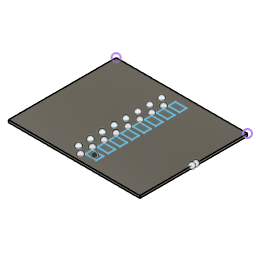
sequence (Autodesk Fusion 360 design; units mm, degrees)
Autodesk Fusion 360 part; units mm, degrees
box "BoxPrimitive1" add length 136 width 166 height 3 placed x (0, -1, 0) y (1, 0, 0) z (0, 0, 1) at (-30, 40, 0)
move_body "Move1" bodies 1 to x (1, 0, 0) y (0, 1, 0) z (0, 0, 1) at (-59.3373, 23.0424, 23.0424)
move_body "Move2" bodies 1 to x (1, 0, 0) y (0, 1, 0) z (0, 0, 1) at (6.3373, 4.9576, -26.0424)
move_body "Move3" bodies 1 to x (1, 0, 0) y (0, 1, 0) z (0, 0, 1) at (0, 0, 3)
sketch "Sketch6" plane through (0, 0, 3) normal (0, 0, 1) x (-1, 0, 0)
  line L0 (83, 68) -> (-83, 68)
  line L1 (-83, 68) -> (-83, -68)
  line L2 (83, -68) -> (83, 68)
  line L3 (11, 54) -> (9, 54)
  line L4 (9, 54) -> (9, 51)
  line L5 (9, 51) -> (11, 51)
  line L6 (11, 51) -> (11, 54)
  line L7 (11, 39) -> (9, 39)
  line L8 (11, 36) -> (11, 39)
  line L9 (9, 39) -> (9, 36)
  line L10 (9, 36) -> (11, 36)
  line L11 (11, 24) -> (9, 24)
  line L12 (11, 21) -> (11, 24)
  line L13 (9, 24) -> (9, 21)
  line L14 (9, 21) -> (11, 21)
  line L15 (11, 9) -> (9, 9)
  line L16 (11, 6) -> (11, 9)
  line L17 (9, 9) -> (9, 6)
  line L18 (9, 6) -> (11, 6)
  line L19 (11, -6) -> (9, -6)
  line L20 (11, -9) -> (11, -6)
  line L21 (9, -6) -> (9, -9)
  line L22 (9, -9) -> (11, -9)
  line L23 (11, -21) -> (9, -21)
  line L24 (11, -24) -> (11, -21)
  line L25 (9, -21) -> (9, -24)
  line L26 (9, -24) -> (11, -24)
  line L27 (11, -36) -> (9, -36)
  line L28 (11, -39) -> (11, -36)
  line L29 (9, -36) -> (9, -39)
  line L30 (9, -39) -> (11, -39)
  line L31 (11, -51) -> (9, -51)
  line L32 (11, -54) -> (11, -51)
  line L33 (9, -51) -> (9, -54)
  line L34 (9, -54) -> (11, -54)
  line L35 (-82, -2.7) -> (-83, -2.7)
  line L36 (-83, 2.3) -> (-82, 2.3)
  line L37 (-82, 2.3) -> (-82, -2.7)
  line L38 (-3, 48) -> (-17, 48)
  line L39 (-17, 48) -> (-17, 57)
  line L40 (-17, 57) -> (-3, 57)
  line L41 (-3, 57) -> (-3, 48)
  line L42 (-17, 42) -> (-3, 42)
  line L43 (-17, 33) -> (-17, 42)
  line L44 (-3, 42) -> (-3, 33)
  line L45 (-3, 33) -> (-17, 33)
  line L46 (-17, 27) -> (-3, 27)
  line L47 (-17, 18) -> (-17, 27)
  line L48 (-3, 27) -> (-3, 18)
  line L49 (-3, 18) -> (-17, 18)
  line L50 (-17, 12) -> (-3, 12)
  line L51 (-17, 3) -> (-17, 12)
  line L52 (-3, 12) -> (-3, 3)
  line L53 (-3, 3) -> (-17, 3)
  line L54 (-17, -3) -> (-3, -3)
  line L55 (-17, -12) -> (-17, -3)
  line L56 (-3, -3) -> (-3, -12)
  line L57 (-3, -12) -> (-17, -12)
  line L58 (-17, -18) -> (-3, -18)
  line L59 (-17, -27) -> (-17, -18)
  line L60 (-3, -18) -> (-3, -27)
  line L61 (-3, -27) -> (-17, -27)
  line L62 (-17, -33) -> (-3, -33)
  line L63 (-17, -42) -> (-17, -33)
  line L64 (-3, -33) -> (-3, -42)
  line L65 (-3, -42) -> (-17, -42)
  line L66 (-17, -48) -> (-3, -48)
  line L67 (-17, -57) -> (-17, -48)
  line L68 (-3, -48) -> (-3, -57)
  line L69 (-3, -57) -> (-17, -57)
  point P0 (0, 60)
  point P1 (10, 52.5)
  point P2 (-10, 52.5)
  point P3 (10, 37.5)
  point P4 (10, 22.5)
  point P5 (10, 7.5)
  point P6 (10, -7.5)
  point P7 (10, -22.5)
  point P8 (10, -37.5)
  point P9 (10, -52.5)
  point P10 (-10, 52.5)
  point P11 (0, 45)
  point P12 (0, 30)
  point P13 (0, 15)
  point P14 (0, -15)
  point P15 (0, -30)
  point P16 (0, -45)
  dimension "d41" = 3
  dimension "d50" = 5
  dimension "d51" = 14
  dimension "d52" = 9
  constraint horizontal L3
  constraint perpendicular L3 L4
  constraint parallel L3 L5
  constraint parallel L4 L6
  constraint horizontal L35
  constraint horizontal L36
  constraint vertical L37
  constraint horizontal L38
  constraint perpendicular L38 L39
  constraint parallel L38 L40
  constraint parallel L39 L41
  constraint coincident P10 P2
  measures "d41" distance of L3.end L4.end
  measures "d50" distance of L35.start L36.end
  measures "d51" distance of L39.end L40.end
  measures "d52" distance of L38.end L39.end
sketch "Sketch4" plane through (0, 0, 3) normal (0, 0, 1) x (-1, 0, 0)
  line L0 (83, 68) -> (-83, 68)
  line L1 (-83, 68) -> (-83, -68)
  line L2 (-83, -68) -> (83, -68)
  line L3 (83, -68) -> (83, 68)
  line L4 (0, 0) -> (0, -20)
  line L5 (0, 0) -> (0, 20)
  line L6 (0, 0) -> (-15, 0)
  line L7 (1, -18.5) -> (-1, -18.5)
  line L8 (-1, -18.5) -> (-1, -21.5)
  line L9 (-1, -21.5) -> (1, -21.5)
  line L10 (1, -21.5) -> (1, -18.5)
  line L11 (1, -18.5) -> (-1, -21.5) construction
  line L12 (-1, -18.5) -> (1, -21.5) construction
  line L13 (-1, 18.5) -> (1, 18.5)
  line L14 (1, 18.5) -> (1, 21.5)
  line L15 (1, 21.5) -> (-1, 21.5)
  line L16 (-1, 21.5) -> (-1, 18.5)
  line L17 (-1, 18.5) -> (1, 21.5) construction
  line L18 (1, 18.5) -> (-1, 21.5) construction
  line L19 (-15, 0) -> (-15, -6)
  line L20 (-15, 0) -> (-15, 6)
  line L21 (-11, -7.5) -> (-19, -7.5)
  line L22 (-19, -7.5) -> (-19, -4.5)
  line L23 (-19, -4.5) -> (-11, -4.5)
  line L24 (-11, -4.5) -> (-11, -7.5)
  line L25 (-11, -7.5) -> (-19, -4.5) construction
  line L26 (-19, -7.5) -> (-11, -4.5) construction
  line L27 (-19, 4.5) -> (-11, 4.5)
  line L28 (-11, 4.5) -> (-11, 7.5)
  line L29 (-11, 7.5) -> (-19, 7.5)
  line L30 (-19, 7.5) -> (-19, 4.5)
  line L31 (-19, 4.5) -> (-11, 7.5) construction
  line L32 (-11, 4.5) -> (-19, 7.5) construction
  point P0 (0, -20)
  point P1 (0, 20)
  point P2 (-15, -6)
  point P3 (-15, 6)
  dimension "d11" = 20
  dimension "d12" = 20
  dimension "d13" = 15
  dimension "d14" = 2
  dimension "d15" = 3
  dimension "d16" = 2
  dimension "d17" = 3
  dimension "d18" = 6
  dimension "d19" = 6
  dimension "d20" = 8
  dimension "d21" = 3
  dimension "d22" = 8
  dimension "d23" = 3
  constraint coincident L4.start L5.start
  constraint vertical L4
  constraint parallel L4 L5
  constraint perpendicular L4 L6
  constraint horizontal L7
  constraint perpendicular L7 L8
  constraint parallel L7 L9
  constraint parallel L8 L10
  constraint coincident L11 P0
  constraint coincident L12 P0
  constraint coincident P0 L4.end
  constraint horizontal L13
  constraint perpendicular L13 L14
  constraint parallel L13 L15
  constraint parallel L14 L16
  constraint coincident L17 P1
  constraint coincident L18 P1
  constraint coincident P1 L5.end
  constraint vertical L19
  constraint perpendicular L6 L20
  constraint horizontal L21
  constraint perpendicular L21 L22
  constraint parallel L21 L23
  constraint parallel L22 L24
  constraint coincident L25 P2
  constraint coincident L26 P2
  constraint coincident P2 L19.end
  constraint horizontal L27
  constraint perpendicular L27 L28
  constraint parallel L27 L29
  constraint parallel L28 L30
  constraint coincident L31 P3
  constraint coincident L32 P3
  constraint coincident P3 L20.end
  measures "d11" distance of L4.start P0
  measures "d12" distance of L4.start P1
  measures "d13" distance of L4.start L6.end
  measures "d14" distance of L8.end L9.end
  measures "d15" distance of L7.end L8.end
  measures "d16" distance of L14.end L15.end
  measures "d17" distance of L13.end L14.end
  measures "d18" distance of L6.end P2
  measures "d19" distance of L6.end P3
  measures "d20" distance of L22.end L23.end
  measures "d21" distance of L21.end L22.end
  measures "d22" distance of L28.end L29.end
  measures "d23" distance of L27.end L28.end
extrude "Extrude1" [suppressed]
